Autodesk Fusion 360 part; units mm, degrees
(part 3 of 3)
  constraint horizontal L839
  constraint vertical L1118
  constraint horizontal L864
  constraint vertical L1040
  constraint horizontal L836
  constraint vertical L890
  constraint horizontal L848
  constraint vertical L1098
  constraint horizontal L870
  constraint vertical L875
  constraint horizontal L867
  constraint vertical L855
  constraint horizontal L879
  constraint vertical L857
  constraint horizontal L884
  constraint vertical L881
  constraint horizontal L843
  constraint vertical L862
  constraint horizontal L856
  constraint vertical L883
  constraint horizontal L1149
  constraint vertical L1159
  constraint horizontal L1124
  constraint vertical L1156
  constraint horizontal L876
  constraint vertical L889
  constraint horizontal L887
  constraint vertical L888
  constraint horizontal L1175
  constraint vertical L961
  constraint horizontal L1029
  constraint vertical L878
  constraint horizontal L1024
  constraint vertical L1010
  constraint horizontal L1056
  constraint vertical L849
  constraint horizontal L1068
  constraint vertical L1182
  constraint horizontal L1186
  constraint vertical L858
  constraint horizontal L1191
  constraint vertical L1177
  constraint horizontal L1197
  constraint vertical L1122
  constraint horizontal L1168
  constraint vertical L1179
  constraint horizontal L1178
  constraint vertical L880
  constraint horizontal L860
  constraint vertical L966
  constraint horizontal L873
  constraint vertical L1000
  constraint horizontal L869
  constraint vertical L835
  constraint horizontal L1138
  constraint vertical L1048
  constraint horizontal L842
  constraint vertical L1127
  constraint horizontal L1154
  constraint vertical L1200
  constraint horizontal L1134
  constraint vertical L1137
  constraint horizontal L1150
  constraint vertical L1166
  constraint horizontal L877
  constraint vertical L983
  constraint horizontal L874
  constraint vertical L1176
  constraint horizontal L926
  constraint vertical L934
  constraint horizontal L909
  constraint vertical L871
  constraint horizontal L972
  constraint vertical L980
  constraint horizontal L922
  constraint vertical L872
  constraint horizontal L950
  constraint vertical L899
  constraint horizontal L906
  constraint vertical L1157
  constraint horizontal L824
  constraint vertical L796
  constraint horizontal L822
  constraint vertical L1140
  constraint horizontal L989
  constraint vertical L975
  constraint horizontal L927
  constraint vertical L834
  constraint horizontal L1045
  constraint vertical L1059
  constraint horizontal L1052
  constraint vertical L863
  constraint horizontal L1069
  constraint vertical L850
  constraint horizontal L1160
  constraint vertical L854
  constraint horizontal L1131
  constraint vertical L1163
  constraint horizontal L1161
  constraint vertical L1145
  constraint horizontal L1143
  constraint vertical L1135
  constraint horizontal L1139
  constraint vertical L1148
  constraint horizontal L1091
  constraint vertical L1079
  constraint horizontal L1099
  constraint vertical L1152
  constraint horizontal L1063
  constraint vertical L1116
  constraint horizontal L1107
  constraint vertical L1121
  constraint horizontal L1011
  constraint vertical L1169
  constraint horizontal L1054
  constraint vertical L865
  constraint horizontal L1065
  constraint vertical L1042
  constraint horizontal L1026
  constraint vertical L1129
  constraint horizontal L954
  constraint vertical L1004
  constraint horizontal L956
  constraint vertical L1123
  constraint horizontal L1058
  constraint vertical L1064
  constraint horizontal L1070
  constraint vertical L837
  constraint horizontal L859
  constraint vertical L1136
  constraint horizontal L833
  constraint vertical L1016
  constraint horizontal L886
  constraint vertical L866
  constraint horizontal L851
  constraint vertical L1164
  constraint horizontal L840
  constraint vertical L1155
  constraint horizontal L1147
  constraint vertical L1022
  constraint horizontal L1117
  constraint vertical L1158
  constraint horizontal L1162
  constraint vertical L958
  constraint horizontal L882
  constraint vertical L845
  constraint horizontal L838
  constraint vertical L1061
  measures "d443" distance of L1 L19
  measures "d445" distance of L0 L596
  measures "d446" distance of L3 L751
extrude "Extrude13" cut sketch "Sketch9" against normal blind 1 draft -30 contours L6 L7 L8 L9 | L10 L11 L12 L13 | L14 L15 L16 L17 | L18 L19 L20 L21 | L22 L23 L24 L25 | L26 L29 L32 L33 | L27 L28 L34 L45 | L30 L31 L36 L44 | L35 L37 L38 L42 | L39 L40 L41 L43 | L46 L49 L57 L80 | L47 L51 L58 L65 | L48 L50 L54 L76 | L52 L53 L70 L74 | L55 L73 L78 L79 | L56 L59 L67 L69 | L60 L61 L81 L84 | L62 L63 L68 L71 | L64 L66 L72 L85 | L75 L77 L82 L83 | L86 L89 L102 L151 | L87 L98 L148 L150 | L88 L96 L99 L101 | L90 L122 L147 L156 | L91 L108 L126 L145 | L92 L94 L143 L160 | L93 L132 L154 L162 | L95 L100 L103 L152 | L97 L107 L134 L153 | L104 L123 L133 L163 | L105 L110 L119 L131 | L106 L111 L113 L114 | L109 L146 L155 L164 | L112 L115 L157 L159 | L116 L158 L161 L165 | L117 L129 L130 L144 | L118 L120 L121 L128 | L124 L125 L140 L149 | L127 L136 L138 L141 | L135 L137 L139 L142 | L166 L170 L179 L183 | L167 L189 L200 L206 | L168 L203 L212 L215 | L169 L175 L177 L181 | L171 L174 L180 L182 | L172 L190 L202 L218 | L173 L208 L209 L224 | L176 L186 L196 L213 | L178 L198 L217 L254 | L184 L201 L205 L211 | L185 L199 L204 L219 | L187 L259 L270 L297 | L188 L191 L242 L304 | L192 L195 L210 L232 | L193 L207 L235 L256 | L194 L317 L320 L323 | L197 L290 L306 L309 | L214 L247 L284 L302 | L216 L243 L249 L322 | L220 L250 L252 L258 | L221 L234 L260 L267 | L222 L238 L263 L264 | L223 L257 L272 L273 | L225 L265 L293 L308 | L226 L231 L239 L288 | L227 L236 L277 L299 | L228 L296 L300 L303 | L229 L253 L255 L279 | L230 L244 L282 L324 | L233 L248 L266 L283 | L237 L240 L262 L274 | L241 L251 L261 L269 | L245 L268 L271 L321 | L246 L278 L289 L313 | L275 L276 L307 L312 | L280 L281 L291 L298 | L285 L286 L292 L311 | L287 L294 L305 L310 | L295 L316 L319 L325 | L301 L314 L315 L318 | L326 L372 L384 L462 | L327 L341 L342 L343 | L328 L329 L330 L332 | L331 L379 L463 L492 | L333 L460 L484 L493 | L334 L335 L337 L612 | L336 L500 L505 L508 | L338 L344 L345 L346 | L339 L529 L535 L554 | L340 L469 L494 L527 | L347 L356 L357 L571 | L348 L352 L575 L577 | L349 L353 L358 L585 | L350 L371 L380 L440 | L351 L513 L595 L605 | L354 L369 L425 L625 | L355 L363 L382 L443 | L359 L367 L432 L592 | L360 L520 L523 L544 | L361 L417 L548 L609 | L362 L524 L564 L565 | L364 L376 L426 L568 | L365 L373 L377 L623 | L366 L378 L381 L383 | L368 L487 L552 L570 | L370 L480 L540 L546 | L374 L498 L525 L578 | L375 L396 L574 L590 | L385 L534 L553 L567 | L386 L421 L430 L468 | L387 L410 L428 L437 | L388 L427 L434 L579 | L389 L397 L541 L559 | L390 L586 L598 L611 | L391 L413 L576 L610 | L392 L393 L476 L485 | L394 L408 L431 L599 | L395 L452 L475 L491 | L398 L450 L459 L471 | L399 L418 L445 L539 | L400 L401 L404 L438 | L402 L406 L409 L411 | L403 L407 L414 L572 | L405 L489 L503 L591 | L412 L486 L588 L596 | L415 L420 L433 L444 | L416 L442 L509 L547 | L419 L423 L435 L521 | L422 L436 L439 L526 | L424 L497 L614 L622 | L429 L447 L604 L608 | L441 L446 L507 L545 | L448 L461 L465 L502 | L449 L467 L473 L543 | L451 L597 L601 L606 | L453 L479 L504 L506 | L454 L455 L481 L490 | L456 L530 L551 L556 | L457 L470 L482 L496 | L458 L478 L495 L624 | L464 L472 L483 L510 | L466 L532 L536 L557 | L474 L477 L533 L549 | L488 L563 L582 L600 | L499 L584 L616 L617 | L501 L516 L517 L522 | L511 L587 L589 L594 | L512 L537 L542 L561 | L514 L580 L593 L607 | L515 L518 L555 L560 | L519 L538 L615 L620 | L528 L602 L613 L621 | L531 L550 L558 L562 | L566 L573 L618 L619 | L569 L581 L583 L603 | L626 L697 L701 L704 | L627 L1204 L1221 L1222 | L628 L733 L769 L772 | L629 L682 L686 L695 | L630 L698 L702 L707 | L631 L700 L705 L706 | L632 L650 L661 L678 | L633 L638 L658 L805 | L634 L644 L821 L1188 | L635 L641 L779 L1172 | L636 L639 L659 L815 | L637 L710 L743 L799 | L640 L647 L784 L788 | L642 L670 L814 L1184 | L643 L725 L742 L809 | L645 L668 L719 L793 | L646 L674 L996 L1096 | L648 L657 L662 L680 | L649 L654 L726 L1125 | L651 L677 L762 L785 | L652 L665 L823 L1076 | L653 L676 L1001 L1077 | L655 L679 L790 L817 | L656 L666 L794 L1201 | L660 L673 L675 L757 | L663 L667 L819 L971 | L664 L669 L917 L1083 | L671 L783 L802 L818 | L672 L795 L808 L944 | L681 L684 L696 L1233 | L683 L690 L692 L1205 | L685 L689 L691 L1226 | L687 L688 L694 L1207 | L693 L1212 L1229 L1237 | L699 L830 L1007 L1208 | L703 L832 L1008 L1009 | L708 L718 L747 L764 | L709 L721 L737 L751 | L711 L744 L759 L760 | L712 L715 L731 L752 | L713 L739 L753 L804 | L714 L727 L942 L988 | L716 L774 L915 L939 | L717 L766 L911 L1006 | L720 L732 L765 L892 | L722 L791 L907 L933 | L723 L745 L758 L976 | L724 L901 L905 L940 | L728 L925 L945 L997 | L729 L740 L746 L754 | L730 L770 L811 L813 | L734 L735 L755 L767 | L736 L803 L902 L943 | L738 L741 L748 L763 | L749 L923 L992 L1217 | L750 L810 L929 L982 | L756 L771 L789 L825 | L761 L797 L800 L1084 | L768 L780 L816 L1119 | L773 L781 L977 L1133 | L775 L941 L946 L969 | L776 L778 L792 L806 | L777 L786 L787 L798 | L782 L820 L993 L1078 | L796 L822 L824 L1140 | L801 L812 L827 L828 | L807 L962 L1171 L1185 | L826 L968 L1002 L1106 | L829 L1202 L1213 L1214 | L831 L1234 L1244 L1245 | L833 L859 L1016 L1136 | L834 L927 L975 L989 | L835 L869 L1048 L1138 | L836 L848 L890 L1098 | L837 L1058 L1064 L1070 | L838 L845 L882 L1061 | L839 L864 L1040 L1118 | L840 L1022 L1147 L1155 | L841 L846 L847 L1080 | L842 L1127 L1154 L1200 | L843 L856 L862 L883 | L844 L853 L861 L1049 | L849 L1010 L1024 L1056 | L850 L854 L1069 L1160 | L851 L866 L886 L1164 | L852 L868 L885 L1112 | L855 L867 L870 L875 | L857 L879 L881 L884 | L858 L1068 L1182 L1186 | L860 L873 L966 L1000 | L863 L1045 L1052 L1059 | L865 L1011 L1054 L1169 | L871 L909 L926 L934 | L872 L922 L972 L980 | L874 L877 L983 L1176 | L876 L887 L888 L889 | L878 L961 L1029 L1175 | L880 L1168 L1178 L1179 | L891 L1027 L1047 L1192 | L893 L897 L924 L937 | L894 L1012 L1013 L1021 | L895 L898 L900 L908 | L896 L913 L948 L949 | L899 L906 L950 L1157 | L903 L919 L936 L952 | L904 L914 L918 L928 | L910 L930 L938 L995 | L912 L932 L947 L1206 | L916 L1034 L1093 L1108 | L920 L931 L1005 L1243 | L921 L1014 L1173 L1194 | L935 L955 L957 L967 | L951 L1025 L1041 L1113 | L953 L970 L978 L981 | L954 L956 L1004 L1123 | L958 L1117 L1158 L1162 | L959 L984 L1183 L1193 | L960 L1092 L1094 L1100 | L963 L1038 L1165 L1174 | L964 L965 L985 L998 | L973 L1020 L1033 L1110 | L974 L1167 L1196 L1198 | L979 L987 L990 L1003 | L986 L991 L994 L999 | L1015 L1043 L1057 L1060 | L1017 L1023 L1028 L1051 | L1018 L1037 L1050 L1189 | L1019 L1046 L1062 L1067 | L1026 L1042 L1065 L1129 | L1030 L1031 L1053 L1066 | L1032 L1036 L1187 L1199 | L1035 L1180 L1190 L1195 | L1039 L1089 L1095 L1115 | L1044 L1055 L1170 L1181 | L1063 L1107 L1116 L1121 | L1071 L1072 L1097 L1114 | L1073 L1120 L1128 L1142 | L1074 L1104 L1105 L1146 | L1075 L1085 L1144 L1151 | L1079 L1091 L1099 L1152 | L1081 L1087 L1088 L1090 | L1082 L1086 L1111 L1141 | L1101 L1102 L1103 L1109 | L1122 L1177 L1191 L1197 | L1124 L1149 L1156 L1159 | L1126 L1130 L1132 L1153 | L1131 L1145 L1161 L1163 | L1134 L1137 L1150 L1166 | L1135 L1139 L1143 L1148 | L1203 L1224 L1225 L1238 | L1209 L1210 L1211 L1220 | L1215 L1216 L1218 L1219 | L1223 L1232 L1236 L1240 | L1227 L1235 L1241 L1242 | L1228 L1230 L1231 L1239 bodies 2 in component "breadboard"
extrude "Extrude9" cut sketch "Sketch9" against normal blind 4 contours L0 L1 L2 L3 bodies 2 in component "breadboard"
sketch "Sketch10" plane through (83, 0, 0) normal (1, 0, 0) x (0, 1, 0) in component "breadboard"
  line L0 (26.5, 6) -> (26.5, 10)
  line L1 (26.5, 10) -> (10, 10)
  line L2 (10, 0) -> (45, 0)
  line L3 (28.5, 10) -> (28.5, 6)
  line L4 (28.5, 6) -> (26.5, 6)
  line L5 (27.5, 5) -> (25.5, 5)
  line L6 (25.5, 0) -> (29.5, 0)
  line L7 (29.5, 0) -> (29.5, 5)
  line L8 (29.5, 5) -> (25.5, 5)
  line L9 (25.5, 5) -> (25.5, 0)
  line L10 (10, 10) -> (10, 0)
  line L11 (45, 0) -> (45, 10)
  line L12 (45, 10) -> (28.5, 10)
  constraint horizontal L5
  constraint horizontal L6
  constraint vertical L7
  constraint horizontal L8
  constraint vertical L9
  constraint coincident L2 L6.start
extrude "Extrude10" add sketch "Sketch10" along normal blind 1 contours L2 L5 L6 L7 L8 L9 bodies 2 in component "breadboard"
sketch "Sketch11" plane through (0, 0, 0) normal (-1, 0, 0) x (0, -1, 0) in component "breadboard"
  line L0 (-26.5, 10) -> (-26.5, 6)
  line L1 (-26.5, 6) -> (-28.5, 6)
  line L2 (-28.5, 6) -> (-28.5, 10)
  line L3 (-28.5, 10) -> (-45, 10)
  line L4 (-45, 0) -> (-10, 0)
  line L5 (-25.5, 5) -> (-29.5, 5)
  line L6 (-29.5, 0) -> (-25.5, 0)
  line L7 (-25.5, 0) -> (-25.5, 5)
  line L8 (-25.5, 5) -> (-29.5, 5)
  line L9 (-29.5, 5) -> (-29.5, 0)
  line L10 (-45, 10) -> (-45, 0)
  line L11 (-10, 0) -> (-10, 10)
  line L12 (-10, 10) -> (-26.5, 10)
  point P0 (-29.5, 0)
  constraint horizontal L6
  constraint vertical L7
  constraint horizontal L8
  constraint vertical L9
  constraint coincident L5.start L7.end
  constraint coincident P0 L6.start
extrude "Extrude11" cut sketch "Sketch11" against normal blind 1 contours L4 L5 L6 L7 L8 L9 bodies 2 in component "breadboard"
sketch "Sketch1 (2)" plane through (0, 0, 10) normal (0, 0, 1) x (-1, 0, 0)
  line L0 (0, 0) -> (-83, 0)
  line L1 (-83, 0) -> (-83, -10)
  line L2 (-83, -10) -> (0, -10)
  line L3 (0, -10) -> (0, 0)
  line L4 (-30, -7.25) -> (-32, -7.25)
  line L5 (-32, -7.25) -> (-32, -5.25)
  line L6 (-32, -5.25) -> (-30, -5.25)
  line L7 (-30, -5.25) -> (-30, -7.25)
  line L8 (-27.5, -5.25) -> (-27.5, -7.25)
  line L9 (-27.5, -7.25) -> (-29.5, -7.25)
  line L10 (-29.5, -5.25) -> (-27.5, -5.25)
  line L11 (-29.5, -7.25) -> (-29.5, -5.25)
  line L12 (-32, -4.75) -> (-32, -2.75)
  line L13 (-32, -2.75) -> (-30, -2.75)
  line L14 (-30, -4.75) -> (-32, -4.75)
  line L15 (-30, -2.75) -> (-30, -4.75)
  line L16 (-27.5, -2.75) -> (-27.5, -4.75)
  line L17 (-27.5, -4.75) -> (-29.5, -4.75)
  line L18 (-29.5, -2.75) -> (-27.5, -2.75)
  line L19 (-29.5, -4.75) -> (-29.5, -2.75)
  line L20 (-25, -7.25) -> (-27, -7.25)
  line L21 (-27, -7.25) -> (-27, -5.25)
  line L22 (-25, -5.25) -> (-25, -7.25)
  line L23 (-27, -5.25) -> (-25, -5.25)
  line L24 (-25, -2.75) -> (-25, -4.75)
  line L25 (-25, -4.75) -> (-27, -4.75)
  line L26 (-27, -2.75) -> (-25, -2.75)
  line L27 (-27, -4.75) -> (-27, -2.75)
  line L28 (-22.5, -7.25) -> (-24.5, -7.25)
  line L29 (-24.5, -7.25) -> (-24.5, -5.25)
  line L30 (-22.5, -5.25) -> (-22.5, -7.25)
  line L31 (-24.5, -5.25) -> (-22.5, -5.25)
  line L32 (-24.5, -2.75) -> (-22.5, -2.75)
  line L33 (-22.5, -2.75) -> (-22.5, -4.75)
  line L34 (-24.5, -4.75) -> (-24.5, -2.75)
  line L35 (-22.5, -4.75) -> (-24.5, -4.75)
  line L36 (-20, -7.25) -> (-22, -7.25)
  line L37 (-22, -7.25) -> (-22, -5.25)
  line L38 (-20, -5.25) -> (-20, -7.25)
  line L39 (-22, -5.25) -> (-20, -5.25)
  line L40 (-20, -2.75) -> (-20, -4.75)
  line L41 (-20, -4.75) -> (-22, -4.75)
  line L42 (-22, -2.75) -> (-20, -2.75)
  line L43 (-22, -4.75) -> (-22, -2.75)
  line L44 (-37.5, -5.25) -> (-35.5, -5.25)
  line L45 (-35.5, -5.25) -> (-35.5, -7.25)
  line L46 (-35.5, -7.25) -> (-37.5, -7.25)
  line L47 (-37.5, -7.25) -> (-37.5, -5.25)
  line L48 (-40, -5.25) -> (-38, -5.25)
  line L49 (-38, -5.25) -> (-38, -7.25)
  line L50 (-40, -7.25) -> (-40, -5.25)
  line L51 (-38, -7.25) -> (-40, -7.25)
  line L52 (-42.5, -5.25) -> (-40.5, -5.25)
  line L53 (-40.5, -5.25) -> (-40.5, -7.25)
  line L54 (-42.5, -7.25) -> (-42.5, -5.25)
  line L55 (-40.5, -7.25) -> (-42.5, -7.25)
  line L56 (-45, -5.25) -> (-43, -5.25)
  line L57 (-43, -5.25) -> (-43, -7.25)
  line L58 (-45, -7.25) -> (-45, -5.25)
  line L59 (-43, -7.25) -> (-45, -7.25)
  line L60 (-47.5, -5.25) -> (-45.5, -5.25)
  line L61 (-45.5, -5.25) -> (-45.5, -7.25)
  line L62 (-47.5, -7.25) -> (-47.5, -5.25)
  line L63 (-45.5, -7.25) -> (-47.5, -7.25)
  line L64 (-47.5, -2.75) -> (-45.5, -2.75)
  line L65 (-45.5, -2.75) -> (-45.5, -4.75)
  line L66 (-47.5, -4.75) -> (-47.5, -2.75)
  line L67 (-45.5, -4.75) -> (-47.5, -4.75)
  line L68 (-45, -2.75) -> (-43, -2.75)
  line L69 (-43, -2.75) -> (-43, -4.75)
  line L70 (-45, -4.75) -> (-45, -2.75)
  line L71 (-43, -4.75) -> (-45, -4.75)
  line L72 (-42.5, -2.75) -> (-40.5, -2.75)
  line L73 (-40.5, -2.75) -> (-40.5, -4.75)
  line L74 (-42.5, -4.75) -> (-42.5, -2.75)
  line L75 (-40.5, -4.75) -> (-42.5, -4.75)
  line L76 (-40, -2.75) -> (-38, -2.75)
  line L77 (-38, -2.75) -> (-38, -4.75)
  line L78 (-40, -4.75) -> (-40, -2.75)
  line L79 (-38, -4.75) -> (-40, -4.75)
  line L80 (-37.5, -2.75) -> (-35.5, -2.75)
  line L81 (-35.5, -2.75) -> (-35.5, -4.75)
  line L82 (-37.5, -4.75) -> (-37.5, -2.75)
  line L83 (-35.5, -4.75) -> (-37.5, -4.75)
  line L84 (-53, -5.25) -> (-51, -5.25)
  line L85 (-51, -5.25) -> (-51, -7.25)
  line L86 (-53, -7.25) -> (-53, -5.25)
  line L87 (-51, -7.25) -> (-53, -7.25)
  line L88 (-53, -2.75) -> (-51, -2.75)
  line L89 (-51, -2.75) -> (-51, -4.75)
  line L90 (-53, -4.75) -> (-53, -2.75)
  line L91 (-51, -4.75) -> (-53, -4.75)
  line L92 (-55.5, -5.25) -> (-53.5, -5.25)
  line L93 (-53.5, -5.25) -> (-53.5, -7.25)
  line L94 (-55.5, -7.25) -> (-55.5, -5.25)
  line L95 (-53.5, -7.25) -> (-55.5, -7.25)
  line L96 (-55.5, -2.75) -> (-53.5, -2.75)
  line L97 (-53.5, -2.75) -> (-53.5, -4.75)
  line L98 (-55.5, -4.75) -> (-55.5, -2.75)
  line L99 (-53.5, -4.75) -> (-55.5, -4.75)
  line L100 (-58, -5.25) -> (-56, -5.25)
  line L101 (-56, -5.25) -> (-56, -7.25)
  line L102 (-58, -7.25) -> (-58, -5.25)
  line L103 (-56, -7.25) -> (-58, -7.25)
  line L104 (-60.5, -5.25) -> (-58.5, -5.25)
  line L105 (-58.5, -5.25) -> (-58.5, -7.25)
  line L106 (-60.5, -7.25) -> (-60.5, -5.25)
  line L107 (-58.5, -7.25) -> (-60.5, -7.25)
  line L108 (-63, -5.25) -> (-61, -5.25)
  line L109 (-61, -5.25) -> (-61, -7.25)
  line L110 (-63, -7.25) -> (-63, -5.25)
  line L111 (-61, -7.25) -> (-63, -7.25)
  line L112 (-63, -2.75) -> (-61, -2.75)
  line L113 (-61, -2.75) -> (-61, -4.75)
  line L114 (-63, -4.75) -> (-63, -2.75)
  line L115 (-61, -4.75) -> (-63, -4.75)
  line L116 (-60.5, -2.75) -> (-58.5, -2.75)
  line L117 (-58.5, -2.75) -> (-58.5, -4.75)
  line L118 (-60.5, -4.75) -> (-60.5, -2.75)
  line L119 (-58.5, -4.75) -> (-60.5, -4.75)
  line L120 (-58, -2.75) -> (-56, -2.75)
  line L121 (-56, -2.75) -> (-56, -4.75)
  line L122 (-58, -4.75) -> (-58, -2.75)
  line L123 (-56, -4.75) -> (-58, -4.75)
  line L124 (-6.5, -5.25) -> (-4.5, -5.25)
  line L125 (-4.5, -5.25) -> (-4.5, -7.25)
  line L126 (-4.5, -7.25) -> (-6.5, -7.25)
  line L127 (-6.5, -7.25) -> (-6.5, -5.25)
  line L128 (-9, -7.25) -> (-9, -5.25)
  line L129 (-7, -5.25) -> (-7, -7.25)
  line L130 (-9, -5.25) -> (-7, -5.25)
  line L131 (-7, -7.25) -> (-9, -7.25)
  line L132 (-11.5, -7.25) -> (-11.5, -5.25)
  line L133 (-11.5, -5.25) -> (-9.5, -5.25)
  line L134 (-9.5, -7.25) -> (-11.5, -7.25)
  line L135 (-9.5, -5.25) -> (-9.5, -7.25)
  line L136 (-14, -5.25) -> (-12, -5.25)
  line L137 (-12, -5.25) -> (-12, -7.25)
  line L138 (-14, -7.25) -> (-14, -5.25)
  line L139 (-12, -7.25) -> (-14, -7.25)
  line L140 (-16.5, -5.25) -> (-14.5, -5.25)
  line L141 (-14.5, -5.25) -> (-14.5, -7.25)
  line L142 (-16.5, -7.25) -> (-16.5, -5.25)
  line L143 (-14.5, -7.25) -> (-16.5, -7.25)
  line L144 (-16.5, -2.75) -> (-14.5, -2.75)
  line L145 (-14.5, -2.75) -> (-14.5, -4.75)
  line L146 (-16.5, -4.75) -> (-16.5, -2.75)
  line L147 (-14.5, -4.75) -> (-16.5, -4.75)
  line L148 (-12, -2.75) -> (-12, -4.75)
  line L149 (-12, -4.75) -> (-14, -4.75)
  line L150 (-14, -2.75) -> (-12, -2.75)
  line L151 (-14, -4.75) -> (-14, -2.75)
  line L152 (-9.5, -2.75) -> (-9.5, -4.75)
  line L153 (-9.5, -4.75) -> (-11.5, -4.75)
  line L154 (-11.5, -2.75) -> (-9.5, -2.75)
  line L155 (-11.5, -4.75) -> (-11.5, -2.75)
  line L156 (-7, -2.75) -> (-7, -4.75)
  line L157 (-7, -4.75) -> (-9, -4.75)
  line L158 (-9, -2.75) -> (-7, -2.75)
  line L159 (-9, -4.75) -> (-9, -2.75)
  line L160 (-4.5, -2.75) -> (-4.5, -4.75)
  line L161 (-4.5, -4.75) -> (-6.5, -4.75)
  line L162 (-6.5, -2.75) -> (-4.5, -2.75)
  line L163 (-6.5, -4.75) -> (-6.5, -2.75)
  line L164 (-68.5, -5.25) -> (-66.5, -5.25)
  line L165 (-66.5, -5.25) -> (-66.5, -7.25)
  line L166 (-66.5, -7.25) -> (-68.5, -7.25)
  line L167 (-68.5, -7.25) -> (-68.5, -5.25)
  line L168 (-71, -5.25) -> (-69, -5.25)
  line L169 (-69, -5.25) -> (-69, -7.25)
  line L170 (-71, -7.25) -> (-71, -5.25)
  line L171 (-69, -7.25) -> (-71, -7.25)
  line L172 (-73.5, -5.25) -> (-71.5, -5.25)
  line L173 (-71.5, -5.25) -> (-71.5, -7.25)
  line L174 (-73.5, -7.25) -> (-73.5, -5.25)
  line L175 (-71.5, -7.25) -> (-73.5, -7.25)
  line L176 (-76, -5.25) -> (-74, -5.25)
  line L177 (-74, -5.25) -> (-74, -7.25)
  line L178 (-76, -7.25) -> (-76, -5.25)
  line L179 (-74, -7.25) -> (-76, -7.25)
  line L180 (-78.5, -5.25) -> (-76.5, -5.25)
  line L181 (-76.5, -5.25) -> (-76.5, -7.25)
  line L182 (-78.5, -7.25) -> (-78.5, -5.25)
  line L183 (-76.5, -7.25) -> (-78.5, -7.25)
  line L184 (-78.5, -2.75) -> (-76.5, -2.75)
  line L185 (-76.5, -2.75) -> (-76.5, -4.75)
  line L186 (-78.5, -4.75) -> (-78.5, -2.75)
  line L187 (-76.5, -4.75) -> (-78.5, -4.75)
  line L188 (-76, -2.75) -> (-74, -2.75)
  line L189 (-74, -2.75) -> (-74, -4.75)
  line L190 (-76, -4.75) -> (-76, -2.75)
  line L191 (-74, -4.75) -> (-76, -4.75)
  line L192 (-73.5, -2.75) -> (-71.5, -2.75)
  line L193 (-71.5, -2.75) -> (-71.5, -4.75)
  line L194 (-73.5, -4.75) -> (-73.5, -2.75)
  line L195 (-71.5, -4.75) -> (-73.5, -4.75)
  line L196 (-71, -2.75) -> (-69, -2.75)
  line L197 (-69, -2.75) -> (-69, -4.75)
  line L198 (-71, -4.75) -> (-71, -2.75)
  line L199 (-69, -4.75) -> (-71, -4.75)
  line L200 (-68.5, -2.75) -> (-66.5, -2.75)
  line L201 (-66.5, -2.75) -> (-66.5, -4.75)
  line L202 (-68.5, -4.75) -> (-68.5, -2.75)
  line L203 (-66.5, -4.75) -> (-68.5, -4.75)
  dimension "d58" = 2
  dimension "d59" = 2
  dimension "d60" = 2
  dimension "d61" = 2
  dimension "d62" = 2
  dimension "d63" = 2
  dimension "d64" = 2
  dimension "d65" = 2
  dimension "d66" = 2
  dimension "d67" = 2
  dimension "d68" = 2
  dimension "d69" = 2
  dimension "d70" = 2
  dimension "d71" = 2
  dimension "d72" = 2
  dimension "d73" = 2
  dimension "d74" = 2
  dimension "d75" = 2
  dimension "d76" = 2
  dimension "d77" = 2
  dimension "d78" = 2
  dimension "d79" = 2
  dimension "d80" = 2
  dimension "d81" = 2
  dimension "d82" = 2
  dimension "d83" = 2
  dimension "d84" = 2
  dimension "d85" = 2
  dimension "d86" = 2
  dimension "d87" = 2
  dimension "d100" = 3.5
  dimension "d116" = 2
  dimension "d117" = 2
  dimension "d118" = 2
  dimension "d119" = 2
  dimension "d120" = 2
  dimension "d121" = 2
  dimension "d122" = 2
  dimension "d123" = 2
  dimension "d124" = 2
  dimension "d125" = 2
  dimension "d126" = 4.5
  dimension "d127" = 2
  dimension "d128" = 2
  dimension "d129" = 2
  dimension "d130" = 2
  dimension "d131" = 2
  dimension "d132" = 2
  dimension "d133" = 2
  dimension "d134" = 2
  dimension "d135" = 2
  dimension "d136" = 2
  dimension "d137" = 4.5
  constraint horizontal L36
  constraint vertical L37
  constraint horizontal L39
  constraint vertical L38
  constraint horizontal L41
  constraint vertical L43
  constraint horizontal L42
  constraint vertical L40
  constraint horizontal L28
  constraint vertical L29
  constraint horizontal L31
  constraint vertical L30
  constraint horizontal L35
  constraint vertical L34
  constraint horizontal L32
  constraint vertical L33
  constraint horizontal L20
  constraint vertical L21
  constraint horizontal L23
  constraint vertical L22
  constraint horizontal L25
  constraint vertical L27
  constraint horizontal L26
  constraint vertical L24
  constraint horizontal L9
  constraint vertical L11
  constraint horizontal L10
  constraint vertical L8
  constraint horizontal L17
  constraint vertical L19
  constraint horizontal L18
  constraint vertical L16
  constraint horizontal L4
  constraint vertical L5
  constraint horizontal L6
  constraint vertical L7
  constraint horizontal L14
  constraint vertical L12
  constraint horizontal L13
  constraint vertical L15
  constraint horizontal L46
  constraint vertical L47
  constraint horizontal L44
  constraint vertical L45
  constraint horizontal L83
  constraint vertical L82
  constraint horizontal L80
  constraint vertical L81
  constraint horizontal L51
  constraint vertical L50
  constraint horizontal L48
  constraint vertical L49
  constraint horizontal L79
  constraint vertical L78
  constraint horizontal L76
  constraint vertical L77
  constraint horizontal L55
  constraint vertical L54
  constraint horizontal L52
  constraint vertical L53
  constraint horizontal L75
  constraint vertical L74
  constraint horizontal L72
  constraint vertical L73
  constraint horizontal L59
  constraint vertical L58
  constraint horizontal L56
  constraint vertical L57
  constraint horizontal L71
  constraint vertical L70
  constraint horizontal L68
  constraint vertical L69
  constraint horizontal L63
  constraint vertical L62
  constraint horizontal L60
  constraint vertical L61
  constraint horizontal L67
  constraint vertical L66
  constraint horizontal L64
  constraint vertical L65
  constraint horizontal L87
  constraint vertical L86
  constraint horizontal L84
  constraint vertical L85
  constraint horizontal L91
  constraint vertical L90
  constraint horizontal L88
  constraint vertical L89
  constraint horizontal L95
  constraint vertical L94
  constraint horizontal L92
  constraint vertical L93
  constraint horizontal L99
  constraint vertical L98
  constraint horizontal L96
  constraint vertical L97
  constraint horizontal L103
  constraint vertical L102
  constraint horizontal L100
  constraint vertical L101
  constraint horizontal L123
  constraint vertical L122
  constraint horizontal L120
  constraint vertical L121
  constraint horizontal L107
  constraint vertical L106
  constraint horizontal L104
  constraint vertical L105
  constraint horizontal L119
  constraint vertical L118
  constraint horizontal L116
  constraint vertical L117
  constraint horizontal L111
  constraint vertical L110
  constraint horizontal L108
  constraint vertical L109
  constraint horizontal L115
  constraint vertical L114
  constraint horizontal L112
  constraint vertical L113
  constraint horizontal L126
  constraint vertical L127
  constraint horizontal L124
  constraint vertical L125
  constraint horizontal L161
  constraint vertical L163
  constraint horizontal L162
  constraint vertical L160
  constraint horizontal L131
  constraint vertical L128
  constraint horizontal L130
  constraint vertical L129
  constraint horizontal L157
  constraint vertical L159
  constraint horizontal L158
  constraint vertical L156
  constraint horizontal L134
  constraint vertical L132
  constraint horizontal L133
  constraint vertical L135
  constraint horizontal L153
  constraint vertical L155
  constraint horizontal L154
  constraint vertical L152
  constraint horizontal L139
  constraint vertical L138
  constraint horizontal L136
  constraint vertical L137
  constraint horizontal L149
  constraint vertical L151
  constraint horizontal L150
  constraint vertical L148
  constraint horizontal L143
  constraint vertical L142
  constraint horizontal L140
  constraint vertical L141
  constraint horizontal L147
  constraint vertical L146
  constraint horizontal L144
  constraint vertical L145
  constraint horizontal L166
  constraint vertical L167
  constraint horizontal L164
  constraint vertical L165
  constraint horizontal L203
  constraint vertical L202
  constraint horizontal L200
  constraint vertical L201
  constraint horizontal L171
  constraint vertical L170
  constraint horizontal L168
  constraint vertical L169
  constraint horizontal L199
  constraint vertical L198
  constraint horizontal L196
  constraint vertical L197
  constraint horizontal L175
  constraint vertical L174
  constraint horizontal L172
  constraint vertical L173
  constraint horizontal L195
  constraint vertical L194
  constraint horizontal L192
  constraint vertical L193
  constraint horizontal L179
  constraint vertical L178
  constraint horizontal L176
  constraint vertical L177
  constraint horizontal L191
  constraint vertical L190
  constraint horizontal L188
  constraint vertical L189
  constraint horizontal L183
  constraint vertical L182
  constraint horizontal L180
  constraint vertical L181
  constraint horizontal L187
  constraint vertical L186
  constraint horizontal L184
  constraint vertical L185
  measures "d58" distance of L36.end L36.start
  measures "d59" distance of L40.end L41.end
  measures "d60" distance of L28.end L28.start
  measures "d61" distance of L34.start L33.end
  measures "d62" distance of L20.end L20.start
  measures "d63" distance of L24.end L25.end
  measures "d64" distance of L9.end L8.end
  measures "d65" distance of L17.end L16.end
  measures "d66" distance of L4.end L4.start
  measures "d67" distance of L12.start L14.start
  measures "d68" distance of L46.end L45.end
  measures "d69" distance of L81.end L82.start
  measures "d70" distance of L50.start L49.end
  measures "d71" distance of L78.start L77.end
  measures "d72" distance of L54.start L53.end
  measures "d73" distance of L73.end L74.start
  measures "d74" distance of L58.start L57.end
  measures "d75" distance of L70.start L69.end
  measures "d76" distance of L62.start L61.end
  measures "d77" distance of L66.start L65.end
  measures "d78" distance of L86.start L85.end
  measures "d79" distance of L89.end L90.start
  measures "d80" distance of L94.start L93.end
  measures "d81" distance of L98.start L97.end
  measures "d82" distance of L101.end L102.start
  measures "d83" distance of L121.end L122.start
  measures "d84" distance of L105.end L106.start
  measures "d85" distance of L118.start L117.end
  measures "d86" distance of L110.start L109.end
  measures "d87" distance of L114.start L113.end
  measures "d100" distance of L5 L45
  measures "d116" distance of L126.end L125.end
  measures "d117" distance of L160.end L161.end
  measures "d118" distance of L128.start L129.end
  measures "d119" distance of L157.end L156.end
  measures "d120" distance of L134.start L132.start
  measures "d121" distance of L152.end L153.end
  measures "d122" distance of L137.end L138.start
  measures "d123" distance of L149.end L148.end
  measures "d124" distance of L142.start L141.end
  measures "d125" distance of L146.start L145.end
  measures "d126" distance of L3 L125
  measures "d127" distance of L165.end L166.end
  measures "d128" distance of L201.end L202.start
  measures "d129" distance of L169.end L170.start
  measures "d130" distance of L198.start L197.end
  measures "d131" distance of L174.start L173.end
  measures "d132" distance of L193.end L194.start
  measures "d133" distance of L178.start L177.end
  measures "d134" distance of L189.end L190.start
  measures "d135" distance of L182.start L181.end
  measures "d136" distance of L185.end L186.start
  measures "d137" distance of L1 L182
extrude "Extrude12" cut sketch "Sketch1 (2)" against normal blind 1 draft -30 contours L4 L5 L6 L7 | L8 L9 L10 L11 | L12 L13 L14 L15 | L16 L17 L18 L19 | L20 L21 L22 L23 | L24 L25 L26 L27 | L28 L29 L30 L31 | L32 L33 L34 L35 | L36 L37 L38 L39 | L40 L41 L42 L43 | L44 L45 L46 L47 | L48 L49 L50 L51 | L52 L53 L54 L55 | L56 L57 L58 L59 | L60 L61 L62 L63 | L64 L65 L66 L67 | L68 L69 L70 L71 | L72 L73 L74 L75 | L76 L77 L78 L79 | L80 L81 L82 L83 | L84 L85 L86 L87 | L88 L89 L90 L91 | L92 L93 L94 L95 | L96 L97 L98 L99 | L100 L101 L102 L103 | L104 L105 L106 L107 | L108 L109 L110 L111 | L112 L113 L114 L115 | L116 L117 L118 L119 | L120 L121 L122 L123 | L124 L125 L126 L127 | L128 L129 L130 L131 | L132 L133 L134 L135 | L136 L137 L138 L139 | L140 L141 L142 L143 | L144 L145 L146 L147 | L148 L149 L150 L151 | L152 L153 L154 L155 | L156 L157 L158 L159 | L160 L161 L162 L163 | L164 L165 L166 L167 | L168 L169 L170 L171 | L172 L173 L174 L175 | L176 L177 L178 L179 | L180 L181 L182 L183 | L184 L185 L186 L187 | L188 L189 L190 L191 | L192 L193 L194 L195 | L196 L197 L198 L199 | L200 L201 L202 L203 bodies 1 in component "breadboard"
copy_body "CopyPasteBodies1" bodies 1 makes body 3
move_body "Move1" bodies 3 to x (-1, 0, 0) y (0, -1, 0) z (0, 0, 1) at (-2, 55, 0)
move_body "Move2" bodies 3 to x (1, 0, 0) y (0, 1, 0) z (0, 0, 1) at (85, 0, 0)
move_face "OffsetFaces1" offset 2 1 faces at (82, 50.6667, 1.3333) on bodies 3
move_face "OffsetFaces2" offset -2 1 faces at (-1, 50.6667, 3.3333) on bodies 3
move_face "OffsetFaces3" offset -2 1 faces at (15.6667, 56, 1.6667) on bodies 3
move_face "OffsetFaces4" offset -2 1 faces at (68.6667, 56, 3.3333) on bodies 3
component "breadboard" placed x (0, 1, 0) y (-1, 0, 0) z (0, 0, 1) at (-35.4067, -29.0665, 3)
